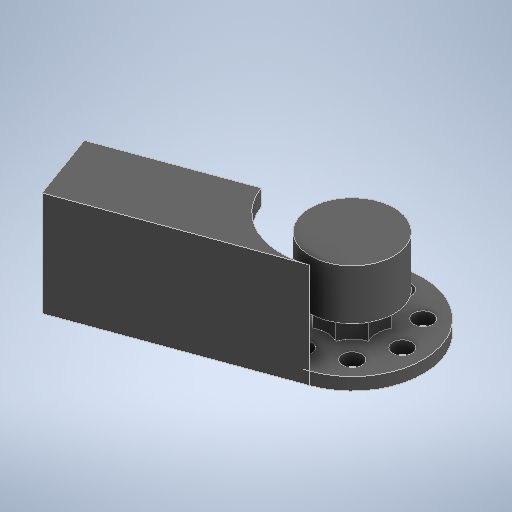
# Autodesk Inventor part: axis
Saved by Autodesk Inventor 2026.1 (Build 301233020, 233B)
## iProperties
Created: 2026-02-27
Part Number: axis
Material: 一般
Document SubType Name: Modeling
Designer: hibik
Density: 1 g/cm^3
Appearance: 既定
Author: hibik
Autodesk Inventor part; units mm, degrees
ref_plane "YZ Plane" through (0, 0, 0) normal (1, 0, 0) x (0, 1, 0)
ref_plane "XZ Plane" through (0, 0, 0) normal (0, 1, 0) x (-1, 0, 0)
ref_plane "XY Plane" through (0, 0, 0) normal (0, 0, 1) x (1, 0, 0)
sketch "スケッチ1" plane through (0, 0, 0) normal (0, 1, 0) x (-1, 0, 0)
  circle A0 centre (0, 0) radius 6 construction
  circle A1 centre (6, 0) radius 1.15
  circle A2 centre (0, 0) radius 8.5
  circle A3 centre (4.2426, 4.2426) radius 1.15
  circle A4 centre (0, 6) radius 1.15
  circle A5 centre (-4.2426, 4.2426) radius 1.15
  circle A6 centre (-6, 0) radius 1.15
  circle A7 centre (-4.2426, -4.2426) radius 1.15
  circle A8 centre (0, -6) radius 1.15
  circle A9 centre (4.2426, -4.2426) radius 1.15
  dimension "d0" = 12
  dimension "d1" = 2.3
  dimension "d2" = 17
  dimension "d5" = 360
  constraints: 9 centre point, 2 coincident, 2 horizontal alignment, 19 other
  measures "d1" diameter of A1
  measures "d2" diameter of A2
extrude "押し出し1" add sketch "スケッチ1" along normal blind 1.5
sketch "スケッチ2" plane through (0, 1.5, 0) normal (0, 1, 0) x (1, 0, 0)
  circle A0 centre (-6, 0) radius 1.15 projected
  circle A1 centre (-6, 0) radius 3
  circle A2 centre (-4.2426, -4.2426) radius 3
  circle A3 centre (0, -6) radius 3
  circle A4 centre (4.2426, -4.2426) radius 3
  circle A5 centre (6, 0) radius 3
  circle A6 centre (4.2426, 4.2426) radius 3
  circle A7 centre (0, 6) radius 3
  circle A8 centre (-4.2426, 4.2426) radius 3
  point P0 (0, 0)
  point P1 (-1.3824, 3.3375)
  point P2 (-3.3375, 1.3824)
  point P3 (-3.3375, -1.3824)
  point P4 (-1.3824, -3.3375)
  point P5 (1.3824, -3.3375)
  point P6 (3.3375, -1.3824)
  point P7 (3.3375, 1.3824)
  point P8 (1.3824, 3.3375)
  dimension "d10" = 6
  dimension "d13" = 360
  constraints: 8 centre point, 1 coincident, 17 other
  measures "d10" diameter of A1
extrude "押し出し2" add sketch "スケッチ2" along normal blind 3 contours A1 A8 A7 A6 A5 A4 A3 A2
sketch "スケッチ3" plane through (0, 4.5, 0) normal (0, 1, 0) x (1, 0, 0)
  circle A0 centre (0, 0) radius 5
  dimension "d17" = 10
  constraints: 1 centre point, 1 coincident
  measures "d17" diameter of A0
extrude "押し出し3" add sketch "スケッチ3" along normal blind 6
sketch "スケッチ4" plane through (0, 0, 0) normal (0, -1, 0) x (1, 0, 0)
  line L0 (0, 0) -> (-23.4923, 8.5505)
  line L1 (-23.4923, 8.5505) -> (0, 0)
  line L2 (-24.2062, 0) -> (13.951, 0) projected
  circle A0 centre (0, 0) radius 5 projected
  line L3 (1.7101, 4.6985) -> (-21.7822, 13.249)
  circle A1 centre (0, 0) radius 8.5 projected
  circle A2 centre (0, 0) radius 8.5 projected
  line L4 (-23.4923, 8.5505) -> (-21.7822, 13.249)
  point P0 (-7.9874, 2.9072)
  point P1 (-4.7492, 7.0495)
  dimension "d20" = 25
  dimension "d21" = 20
  constraints: 8 end point, 1 parallel, 1 perpendicular, 3 other
  measures "d20" distance of L0.start L0.end
  measures "d21" angle of L0 L2
extrude "押し出し4" add sketch "スケッチ4" against normal up to surface (4.5 mm away) contours L0 L4 L3 A1
sketch "スケッチ5" plane through (0, 0, 0) normal (0, -1, 0) x (1, 0, 0)
  line L0 (-4.7492, 7.0495) -> (-21.7822, 13.249) projected
  arc A0 (-7.9874, 2.9072) -> (-4.7492, 7.0495) centre (0, 0) ccw projected
  line L1 (-21.7822, 13.249) -> (-20.5851, 16.5379)
  line L2 (-20.5851, 16.5379) -> (2.9072, 7.9874)
  constraints: 4 end point, 2 perpendicular, 1 point on circle, 1 tangent
extrude "押し出し5" add sketch "スケッチ5" against normal up to surface (10.5 mm away)
sketch "スケッチ6" plane through (-20.5851, 10.5, 16.5379) normal (0, 1, 0) x (0.9396926, 0, -0.3420201)
  arc A0 (16.5, 8.5) -> (18.1261, 3.5) centre (25, 8.5) ccw projected
  line L0 (0, 8.5) -> (16.5, 8.5) projected
  line L1 (0, 3.5) -> (0, 8.5) projected
  line L2 (18.1261, 3.5) -> (0, 3.5) projected
  arc A1 (18.1261, 3.5) -> (25, 0) centre (25, 8.5) ccw projected
  line L3 (0, 3.5) -> (18.1261, 3.5) projected
  line L4 (0, 0) -> (0, 3.5) projected
  line L5 (25, 0) -> (0, 0) projected
  point P0 (0, 3.5)
  point P1 (18.1261, 3.5)
extrude "押し出し6" add sketch "スケッチ6" along normal blind 2
